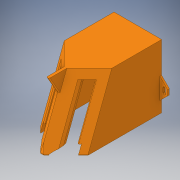
# Autodesk Inventor part: Diverter--v3
Saved by Autodesk Inventor 2019 (Build 230136000, 136)
## iProperties
Created: 2019-02-09
Part Number: Diverter--v3
Material: Generic
Document SubType Name: Modeling
Designer: scigu
Density: 1 g/cm^3
Appearance: Orange
Author: scigu
Autodesk Inventor part; units mm, degrees
ref_plane "YZ Plane" through (0, 0, 0) normal (1, 0, 0) x (0, 1, 0)
ref_plane "XY Plane" through (0, 0, 0) normal (0, 0, 1) x (1, 0, 0)
sketch "Sketch1" plane through (0, 0, 0) normal (0, 1, 0) x (-1, 0, 0)
  line L0 (0, 0) -> (0, 108.0262) construction
  line L1 (0, 0) -> (108.0262, 0) construction
  line L2 (0, 0) -> (-25.4, 0) construction
  line L3 (0, 0) -> (25.4, 0) construction
  line L4 (-25.4, 0) -> (25.4, 0) construction
  line L5 (25.4, 0) -> (25.4, 108.0262) construction
  line L6 (25.4, 108.0262) -> (-25.4, 108.0262) construction
  line L7 (-25.4, 108.0262) -> (-25.4, 0) construction
  line L8 (0, 108.0262) -> (25.4, 82.6262) construction
  line L9 (0, 108.0262) -> (35.921, 108.0262) construction
  line L10 (0, 108.0262) -> (-25.4, 82.6262) construction
  line L11 (0, 108.0262) -> (35.921, 108.0262) construction
  dimension "d0" = 108.0262
  dimension "d1" = 90
  dimension "d2" = 25.4
  dimension "d3" = 180
  dimension "d4" = 50.8
  dimension "d5" = 108.0262
  dimension "d6" = 45
  dimension "d7" = 135
  constraints: 24 end point, 6 horizontal, 4 equal length, 2 parallel, 2 point on line, 1 perpendicular, 1 vertical
  measures "d0" distance of L0.start L0.end
  measures "d1" angle of L1 L0
  measures "d2" distance of L0.start L2.end
  measures "d3" angle of L2 L3
  measures "d4" distance of L6.end L5.end
  measures "d5" distance of L5.end L4.end
  measures "d6" angle of L8 L9
  measures "d7" angle of L10 L11
ref_plane "Work Plane1" through (0, 0, 108.0262) normal (0.6830127, 0.258819, 0.6830127) x (0.7071068, 0, -0.7071068)
ref_plane "Work Plane2" through (0, 0, 108.0262) normal (0.6830127, -0.258819, -0.6830127) x (-0.7071068, 0, -0.7071068)
sketch "Sketch2" plane through (0, 0, 108.0262) normal (0.6830127, 0.258819, 0.6830127) x (0.7071068, 0, -0.7071068)
  line L0 (0, 0) -> (127, 0)
  line L1 (127, 0) -> (127, 127)
  line L2 (127, 127) -> (0, 127)
  line L3 (0, 127) -> (0, 0)
  point P0 (76.3861, 19.7702)
  dimension "d10" = 127
  dimension "d11" = 127
  constraints: 8 end point, 2 parallel, 1 horizontal, 1 perpendicular
  measures "d10" distance of L2.end L1.end
  measures "d11" distance of L1.end L0.end
extrude "Extrusion1" add sketch "Sketch2" along normal blind 3
sketch "Sketch3" plane through (0, 0, 108.0262) normal (0.6830127, -0.258819, -0.6830127) x (-0.7071068, 0, -0.7071068)
  line L0 (0, 0) -> (0, 32.87) projected
  line L1 (0, 0) -> (127, 0)
  line L2 (127, 0) -> (127, 127)
  line L3 (127, 127) -> (0, 127)
  line L4 (0, 127) -> (0, 0)
  point P0 (76.3861, 19.7702)
  dimension "d14" = 127
  dimension "d15" = 127
  constraints: 8 end point, 2 parallel, 1 horizontal, 1 perpendicular
  measures "d14" distance of L3.end L2.end
  measures "d15" distance of L2.end L1.end
extrude "Extrusion2" add sketch "Sketch3" against normal blind 3
sketch "Sketch4" plane through (0, 0, 0) normal (0, 0, 1) x (1, 0, 0)
  line L0 (0, 0) -> (-25.4, 0) construction
  line L1 (0, 0) -> (-89.8026, 0) construction
  line L2 (0, 0) -> (25.4, 0) construction
  line L3 (-25.4, 0) -> (-27.4, 0)
  line L4 (-27.4, 0) -> (-27.4, 73.0758)
  line L5 (-27.4, 73.0758) -> (-25.4, 73.0758)
  line L6 (-25.4, 73.0758) -> (-25.4, 0)
  line L7 (-23.2426, 122.6726) -> (0, 0) construction
  line L8 (0, 0) -> (25.4, 0) construction
  line L9 (0, 0) -> (89.8026, 0) construction
  line L10 (0, 0) -> (25.4, 0) construction
  line L11 (25.4, 0) -> (27.4, 0)
  line L12 (27.4, 0) -> (27.4, 73.0758)
  line L13 (27.4, 73.0758) -> (25.4, 73.0758)
  line L14 (25.4, 73.0758) -> (25.4, 0)
  line L15 (25.4, 73.0758) -> (-25.4, 73.0758)
  line L16 (-25.4, 73.0758) -> (-25.4, 71.0758)
  line L17 (-25.4, 71.0758) -> (25.4, 71.0758)
  line L18 (25.4, 71.0758) -> (25.4, 73.0758)
  line L19 (-27.4, 0) -> (-94.5199, 0)
  line L20 (-94.5199, 0) -> (-94.5199, 116.3337)
  line L21 (-94.5199, 116.3337) -> (-27.4, 116.3337)
  line L22 (-27.4, 116.3337) -> (-27.4, 0)
  line L23 (-27.4, 73.0758) -> (27.4, 73.0758)
  line L24 (27.4, 73.0758) -> (27.4, 116.3337)
  line L25 (27.4, 116.3337) -> (-27.4, 116.3337)
  line L26 (-27.4, 116.3337) -> (-27.4, 73.0758)
  line L27 (27.4, 0) -> (105.8301, 0)
  line L28 (105.8301, 0) -> (105.8301, 116.3337)
  line L29 (105.8301, 116.3337) -> (27.4, 116.3337)
  line L30 (27.4, 116.3337) -> (27.4, 0)
  line L31 (105.8301, 0) -> (-94.5199, 0)
  line L32 (-94.5199, 0) -> (-94.5199, -3.4883)
  line L33 (-94.5199, -3.4883) -> (105.8301, -3.4883)
  line L34 (105.8301, -3.4883) -> (105.8301, 0)
  line L35 (-94.5199, 116.3337) -> (105.8301, 116.3337)
  line L36 (105.8301, 116.3337) -> (105.8301, 158.6024)
  line L37 (105.8301, 158.6024) -> (-94.5199, 158.6024)
  line L38 (-94.5199, 158.6024) -> (-94.5199, 116.3337)
  point P0 (-2.4495, 0)
  point P1 (2.4495, 0)
  dimension "d18" = 25.4
  dimension "d19" = 180
  dimension "d20" = 2
  dimension "d21" = 73.0758
  dimension "d22" = 25.4
  dimension "d23" = 0
  dimension "d24" = 2
  dimension "d25" = 73.0758
  dimension "d26" = 50.8
  dimension "d27" = 2
  constraints: 72 end point, 16 parallel, 10 horizontal, 8 perpendicular, 4 collinear, 2 point on line
  measures "d18" distance of L0.start L0.end
  measures "d19" angle of L2 L0
  measures "d20" distance of L4.end L5.end
  measures "d21" distance of L3.end L4.end
  measures "d22" distance of L0.start L2.end
  measures "d23" distance between parallel lines of L8 L10
  measures "d24" distance of L13.end L12.end
  measures "d25" distance of L12.end L11.end
  measures "d26" distance of L17.end L16.end
  measures "d27" distance of L16.end L15.end
extrude "Extrusion3" add sketch "Sketch4" along normal up to next contours L3 L4 L5 L6 | L6 L15 L14 L17 | L14 L13 L12 L11
extrude "Extrusion4" cut sketch "Sketch4" along normal through all both and the other way through all contours L31 L11 L27 L34 L33 L32 L19 L3 | L19 L20 L21 L22 L4 | L22 L25 L24 L13 L15 L5 | L12 L24 L29 L28 L27 | L21 L38 L37 L36 L29 L25
ref_plane "Work Plane3" through (-2.1962, 73.0915, 82.5252) normal (0.7304065, -0.2420251, -0.6386941) x (0, -0.9351131, 0.3543493)
sketch "Sketch6" plane through (-2.1962, 73.0915, 82.5252) normal (0.7304065, -0.2420251, -0.6386941) x (0, -0.9351131, 0.3543493)
  line L0 (66.5461, -3) -> (77.3851, -3) projected
  line L1 (66.5461, -3) -> (-70.956, -3)
  line L2 (-70.956, -3) -> (-70.956, -37.0198)
  line L3 (-70.956, -37.0198) -> (66.5461, -37.0198)
  line L4 (66.5461, -37.0198) -> (66.5461, -3)
  point P0 (39.1061, 73.7833)
  point P1 (-83.645, 0)
  point P2 (-45.5636, -3)
  constraints: 8 end point, 2 parallel, 1 horizontal, 1 perpendicular
extrude "Extrusion5" cut sketch "Sketch6" along normal through all both and the other way through all
ref_plane "Work Plane4" through (2.1962, 73.0915, 82.5252) normal (0.7304065, 0.2420251, 0.6386941) x (0, -0.9351131, 0.3543493)
sketch "Sketch7" plane through (2.1962, 73.0915, 82.5252) normal (0.7304065, 0.2420251, 0.6386941) x (0, -0.9351131, 0.3543493)
  line L0 (66.5461, -3) -> (77.3851, 0) projected
  line L1 (66.5461, -3) -> (-54.8375, -3)
  line L2 (-54.8375, -3) -> (-54.8375, -46.8131)
  line L3 (-54.8375, -46.8131) -> (66.5461, -46.8131)
  line L4 (66.5461, -46.8131) -> (66.5461, -3)
  point P0 (39.1061, 73.7833)
  point P1 (77.3851, 0)
  point P2 (76.2371, -3)
  constraints: 8 end point, 2 parallel, 1 horizontal, 1 perpendicular, 1 other
extrude "Extrusion6" cut sketch "Sketch7" along normal through all both and the other way through all
sketch "Sketch8" plane through (0, 0, 0) normal (1, 0, 0) x (0, 1, 0)
  line L0 (0, 108.0262) -> (0, 80.6262) construction
  line L1 (0, 0) -> (0, 108.0262) construction
  line L2 (0, 0) -> (108.0262, 0) construction
  line L3 (0, 108.0262) -> (-23.3345, 84.6917) construction
  circle A0 centre (-23.3345, 84.6917) radius 33
  dimension "d38" = 108.0262
  dimension "d39" = 90
  dimension "d40" = 33
  dimension "d41" = 45
  constraints: 6 end point, 1 coincident, 1 horizontal, 1 perpendicular, 1 vertical, 3 other
  measures "d38" distance of L1.start L0.start
  measures "d39" angle of L2 L1
  measures "d40" distance of L0.start L3.end
  measures "d41" angle of L3 L1
extrude "Extrusion7" cut sketch "Sketch8" along normal mid plane 44
sketch "Sketch9" plane through (25.4, 0, 0) normal (0, -1, 0) x (1, 0, 0)
  line L0 (2, 0) -> (2, 80.6262) projected
  line L1 (2, 84.7243) -> (2, 57.3274) projected
  line L2 (2, 80.6262) -> (2, 84.7243)
  line L3 (-3.4, 90.1243) -> (2, 84.7243) projected
  line L4 (2, 84.7243) -> (-3.4, 90.1243)
  line L5 (-3.4, 86.0262) -> (-3.4, 82.3939) projected
  line L6 (-3.4, 90.1243) -> (-3.4, 86.0262)
  line L7 (-3.4, 86.0262) -> (2, 80.6262)
  line L8 (-50.8, 82.6262) -> (-52.8, 80.6262) projected
  line L9 (-52.8, 80.6262) -> (-47.4, 86.0262)
  line L10 (-47.4, 86.0262) -> (-47.4, 90.1243) projected
  line L11 (-47.4, 86.0262) -> (-47.4, 90.1243)
  line L12 (-47.4, 90.1243) -> (-52.8, 84.7243)
  line L13 (-52.8, 84.7243) -> (-52.8, 80.6262)
  line L14 (-23.351, 110.0752) -> (-20.4987, 107.223) projected
  line L15 (-25.4, 108.0262) -> (-20.4987, 107.223)
  line L16 (-20.4987, 107.223) -> (-27.4956, 114.2199)
  ellipse E0 centre (74.4232, 84.6917) end of major axis (251.6893, 91.0471) minor radius 32.403 (-25.4, 108.0262) -> (-30.3013, 107.223) ccw projected
  line L17 (-25.4, 108.0262) -> (-25.4, 108.0262)
  line L18 (-25.4, 108.0262) -> (-25.4, 108.0262)
  line L19 (-30.3013, 107.223) -> (-25.4, 112.1243)
  line L20 (-25.4, 108.0262) -> (-23.351, 110.0752) projected
  line L21 (-25.4, 108.0262) -> (-27.449, 110.0752) projected
  line L22 (-23.351, 110.0752) -> (-27.449, 110.0752)
  point P0 (-25.4, 0)
  constraints: 28 end point, 4 parallel, 3 collinear, 2 point on line, 1 horizontal, 1 perpendicular, 1 vertical, 1 other
extrude "Extrusion8" add sketch "Sketch9" against normal up to next contours L1 L7 L6 L3 | L8 L13 L12 L10 L9
sketch "Sketch11" plane through (0, 0, 0) normal (1, 0, 0) x (0, 1, 0)
  line L0 (11.5911, 108.0262) -> (0, 108.0262) projected
  line L1 (11.5911, 108.0262) -> (0, 108.0262)
  line L2 (0, 108.0262) -> (0.7765, 110.0752) projected
  line L3 (0, 108.0262) -> (0.7765, 110.0752)
  line L4 (0.7765, 110.0752) -> (11.5911, 108.0262)
  point P0 (0, 0)
  constraints: 6 end point, 1 collinear, 1 horizontal
extrude "Extrusion9" add sketch "Sketch11" against normal up to surface starts on plane at (0, 0, 108.0262) facing (0.7071068, 0, 0.7071068) surface through (-23.2426, 122.6726, 84.7836) normal (-0.7071068, 0, 0.7071068)
extrude "Extrusion10" add sketch "Sketch9" along normal up to surface contours L14 L15 L20 surface through (0, 0, 108.0262) normal (0.1830127, -0.9659258, 0.1830127)
extrude "Extrusion11" add sketch "Sketch9" along normal up to surface contours E0 L19 L21 surface through (-89.8026, 0, 18.2236) normal (-0.1830127, -0.9659258, 0.1830127)
extrude "Extrusion12" add sketch "Sketch9" along normal up to surface contours L20 L21 L22 surface through (0, 0.7765, 110.0752) normal (0, -0.9351131, 0.3543493)
sketch "Sketch12" plane through (0, 0, 0) normal (0, 0, -1) x (-1, 0, 0)
  line L0 (0, 0) -> (11, 0) construction
  line L1 (0, 0) -> (-11, 0) construction
  line L2 (-2.049, 0) -> (2.049, 0) construction
  line L3 (11, 0) -> (19, 0)
  line L4 (19, 0) -> (19, 63.5)
  line L5 (19, 63.5) -> (11, 63.5)
  line L6 (11, 63.5) -> (11, 0)
  line L7 (-11, 0) -> (-19, 0)
  line L8 (-19, 0) -> (-19, 63.5)
  line L9 (-19, 63.5) -> (-11, 63.5)
  line L10 (-11, 63.5) -> (-11, 0)
  dimension "d54" = 11
  dimension "d55" = 11
  dimension "d56" = 8
  dimension "d57" = 63.5
  dimension "d58" = 8
  dimension "d59" = 63.5
  constraints: 20 end point, 4 parallel, 3 horizontal, 2 perpendicular, 1 collinear
  measures "d54" distance of L0.start L0.end
  measures "d55" distance of L0.start L1.end
  measures "d56" distance of L5.end L4.end
  measures "d57" distance of L4.end L3.end
  measures "d58" distance of L8.end L9.end
  measures "d59" distance of L7.end L8.end
extrude "Extrusion13" cut sketch "Sketch12" against normal through all
sketch "Sketch13" plane through (0, 0, 0) normal (0, 0, -1) x (-1, 0, 0)
  line L0 (0, 0) -> (0, 25.4) construction
  line L1 (0, 0) -> (25.4, 0) construction
  line L2 (0, 25.4) -> (27.4, 25.4) construction
  line L3 (27.4, 0) -> (27.4, 73.0758) construction
  line L4 (27.4, 25.4) -> (27.4, 33.02) construction
  line L5 (27.4, 25.4) -> (32.48, 25.4) construction
  line L6 (27.4, 25.4) -> (32.48, 25.4) construction
  line L7 (27.4, 33.02) -> (36.29, 33.02)
  line L8 (36.29, 33.02) -> (36.29, 17.78)
  line L9 (36.29, 17.78) -> (27.4, 17.78)
  line L10 (27.4, 17.78) -> (27.4, 33.02)
  line L11 (32.48, 22.86) -> (32.48, 27.94) construction
  line L12 (19, 63.5) -> (19, 9.6586) projected
  line L13 (33.98, 22.86) -> (33.98, 27.94)
  line L14 (30.98, 27.94) -> (30.98, 22.86)
  arc A0 (30.98, 22.86) -> (33.98, 22.86) centre (32.48, 22.86) ccw
  arc A1 (33.98, 27.94) -> (30.98, 27.94) centre (32.48, 27.94) ccw
  line L15 (32.48, 25.4) -> (37.56, 25.4) construction
  line L16 (0, 25.4) -> (-27.4, 25.4) construction
  line L17 (-27.4, 0) -> (-27.4, 73.0758) construction
  line L18 (-27.4, 25.4) -> (-27.4, 33.02) construction
  line L19 (-27.4, 25.4) -> (-32.48, 25.4) construction
  line L20 (-27.4, 25.4) -> (-32.48, 25.4) construction
  line L21 (-27.4, 33.02) -> (-36.29, 33.02)
  line L22 (-36.29, 33.02) -> (-36.29, 17.78)
  line L23 (-36.29, 17.78) -> (-27.4, 17.78)
  line L24 (-27.4, 17.78) -> (-27.4, 33.02)
  line L25 (-32.48, 22.86) -> (-32.48, 27.94) construction
  line L26 (-33.98, 22.86) -> (-33.98, 27.94)
  line L27 (-30.98, 27.94) -> (-30.98, 22.86)
  arc A2 (-33.98, 22.86) -> (-30.98, 22.86) centre (-32.48, 22.86) ccw
  arc A3 (-30.98, 27.94) -> (-33.98, 27.94) centre (-32.48, 27.94) ccw
  line L28 (-32.48, 25.4) -> (-37.56, 25.4) construction
  dimension "d62" = 25.4
  dimension "d63" = 90
  dimension "d64" = 27.4
  dimension "d65" = 90
  dimension "d66" = 7.62
  dimension "d67" = 90
  dimension "d68" = 5.08
  dimension "d69" = 0
  dimension "d70" = 8.89
  dimension "d71" = 15.24
  dimension "d72" = 2.54
  dimension "d73" = 90
  dimension "d74" = 3
  constraints: 58 end point, 16 symmetric about line, 8 point on circle, 5 horizontal, 4 centre point, 4 parallel, 4 tangent, 3 equal length, 3 perpendicular, 1 midpoint, 1 vertical, 2 other
  measures "d62" distance of L0.start L0.end
  measures "d63" angle of L1 L0
  measures "d64" distance of L0.end L2.end
  measures "d65" angle of L0 L2
  measures "d66" distance of L2.end L4.end
  measures "d67" angle of L4 L2
  measures "d68" distance of L2.end L5.end
  measures "d69" distance between parallel lines of L5 L6
  measures "d70" distance of L8.end L9.end
  measures "d71" distance of L7.end L8.end
  measures "d72" distance of L6.end L11.end
  measures "d73" angle of L15 L11
  measures "d74" diameter of A1
extrude "Extrusion14" add sketch "Sketch13" against normal blind 2
chamfer "Chamfer1" distance 4.445 angle 45 8 edges at (36.29, 33.02, 1) (27.4, 33.02, 1) (36.29, 17.78, 1) (27.4, 17.78, 1) (-27.4, 33.02, 1) (-36.29, 33.02, 1) (-36.29, 17.78, 1) (-27.4, 17.78, 1)
chamfer "Chamfer2" distance 1.905 angle 45 4 edges at (19, 36.3749, 79.6347) (11, 34.9533, 88.1734) (-11, 34.9533, 88.1734) (-19, 36.3749, 79.6347)
sketch "Sketch14" plane through (0, 0, 0) normal (1, 0, 0) x (0, 1, 0)
  line L0 (73.0758, 84.7274) -> (11.5911, 108.0262) projected
  line L1 (73.0758, 84.7274) -> (73.0758, 103.7774)
  line L2 (73.0758, 84.7274) -> (92.1258, 84.7274) construction
  line L3 (73.0758, 103.7774) -> (53.155, 92.2761)
  line L4 (73.0758, 103.7774) -> (96.0783, 103.7774) construction
  line L5 (73.0758, 84.7274) -> (73.0758, 57.3274) projected
  line L6 (53.155, 92.2761) -> (73.0758, 84.7274)
  point P0 (0, 0)
  dimension "d83" = 19.05
  dimension "d84" = 90
  dimension "d85" = 150
  constraints: 10 end point, 2 equal length, 2 horizontal, 1 point on line, 1 vertical
  measures "d83" distance of L0.start L1.end
  measures "d84" angle of L2 L1
  measures "d85" angle of L3 L4
extrude "Extrusion15" add sketch "Sketch14" along normal mid plane 3
sketch "Sketch15" plane through (0, 53.155, 92.2761) normal (0, -0.3543493, -0.9351131) x (-1, 0, 0)
  line L0 (1.5, 0) -> (0, 0) projected
  line L1 (0, 21.3031) -> (1.5, 21.3031) projected
  line L2 (0, 0) -> (1.5, 0)
  line L3 (1.5, 0) -> (1.5, 21.3031)
  line L4 (1.5, 21.3031) -> (0, 21.3031)
  line L5 (0, 21.3031) -> (0, 0)
  point P0 (0, -17.008)
  constraints: 8 end point, 2 parallel, 1 horizontal, 1 perpendicular
extrude "Extrusion16" add sketch "Sketch15" along normal up to next
sketch "Sketch16" plane through (1.5, 73.0758, 84.7274) normal (0, -0.3543493, -0.9351131) x (-1, 0, 0)
  line L0 (1.5, 0) -> (1.5, -21.3031) projected
  line L1 (1.5, -21.3031) -> (0, -21.3031) projected
  line L2 (1.5, 0) -> (0, 0)
  line L3 (0, 0) -> (0, -21.3031)
  line L4 (0, -21.3031) -> (1.5, -21.3031)
  line L5 (1.5, -21.3031) -> (1.5, 0)
  point P0 (1.5, -38.3111)
  constraints: 8 end point, 2 parallel, 1 horizontal, 1 perpendicular
extrude "Extrusion17" add sketch "Sketch16" along normal up to next
sketch "Sketch17" plane through (0, 73.0758, 84.7274) normal (0, 0.9351131, -0.3543493) x (1, 0, 0)
  line L0 (1.5, 1.4027) -> (0, 0) projected
  line L1 (0, 0) -> (1.5, 1.4027)
  line L2 (1.5, 0) -> (1.5, 1.4027) projected
  line L3 (1.5, 1.4027) -> (1.5, 0)
  line L4 (1.5, 0) -> (0, 0)
  line L5 (0, 0) -> (-1.5, 0) projected
  line L6 (-1.5, 0) -> (-1.5, 1.4027) projected
  line L7 (0, 0) -> (-1.5, 0)
  line L8 (-1.5, 0) -> (-1.5, 1.4027)
  line L9 (-1.5, 1.4027) -> (0, 0)
  point P0 (0, 105.124)
  constraints: 12 end point, 3 collinear, 1 horizontal, 1 perpendicular
extrude "Extrusion18" add sketch "Sketch17" along normal up to surface surface through (25.4, 73.0758, 0) normal (0, 1, 0)
chamfer "Chamfer3" distance 1 angle 45 2 edges at (1.5, 63.1154, 98.0267) (-1.5, 63.1154, 98.0267)
body "Solid1"
